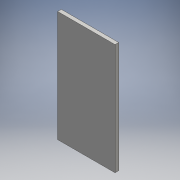
# Autodesk Inventor part: gora
Saved by Autodesk Inventor 2016 SP1 (Build 200210100, 210)
## iProperties
Created: 2019-02-20
Part Number: gora
Material: Ogólny
Document SubType Name: Modeling
Designer: Maciek
Density: 1 g/cm^3
Appearance: Domyślna
Author: Maciek
Autodesk Inventor part; units mm, degrees
ref_plane "YZ Plane" through (0, 0, 0) normal (1, 0, 0) x (0, 1, 0)
ref_plane "XZ Plane" through (0, 0, 0) normal (0, 1, 0) x (-1, 0, 0)
ref_plane "XY Plane" through (0, 0, 0) normal (0, 0, 1) x (1, 0, 0)
sketch "Szkic1" plane through (0, 0, 0) normal (0, 1, 0) x (-1, 0, 0)
  line L0 (0, 0) -> (23.5, 0)
  line L1 (23.5, 0) -> (23.5, 45.5)
  line L2 (23.5, 45.5) -> (0, 45.5)
  line L3 (0, 45.5) -> (0, 0)
  dimension "d0" = 23.5
  dimension "d1" = 45.5
  constraints: 8 end point, 2 parallel, 1 horizontal, 1 perpendicular
  measures "d0" distance of L2.end L1.end
  measures "d1" distance of L1.end L0.end
extrude "Wyciągnięcie proste1" add sketch "Szkic1" along normal blind 1.5
sketch "Szkic2" plane through (0, 1.5, 0) normal (0, 1, 0) x (1, 0, 0)
  line L0 (-23.5, 0) -> (-23.5, -45.5) construction
  line L1 (-23.5, -45.5) -> (-22, -45.5) construction
  line L2 (-23.5, -45.5) -> (0, -45.5) construction
  line L3 (-22, -45.5) -> (-22, -44) construction
  line L4 (-22, -44) -> (-1.5, -44)
  line L5 (-1.5, -44) -> (-1.5, -1.5)
  line L6 (-1.5, -1.5) -> (-22, -1.5)
  line L7 (-22, -1.5) -> (-22, -44)
  line L8 (-22, -44) -> (-22, -42.5) construction
  line L9 (-22, -42.5) -> (-20.5, -42.5) construction
  line L10 (-1.5, -1.5) -> (-3, -1.5) construction
  line L11 (-3, -1.5) -> (-3, -3) construction
  line L12 (-20.5, -42.5) -> (-3, -42.5)
  line L13 (-3, -42.5) -> (-3, -3)
  line L14 (-3, -3) -> (-20.5, -3)
  line L15 (-20.5, -3) -> (-20.5, -42.5)
  point P0 (0, 0)
  dimension "d4" = 1.5
  dimension "d5" = 1.5
  dimension "d6" = 20.5
  dimension "d7" = 42.5
  dimension "d8" = 1.5
  dimension "d9" = 1.5
  dimension "d10" = 1.5
  dimension "d11" = 1.5
  constraints: 28 end point, 4 parallel, 4 perpendicular, 3 point on line, 2 horizontal, 1 vertical
  measures "d4" distance of L0.end L1.end
  measures "d5" distance of L1.end L3.end
  measures "d6" distance of L6.end L5.end
  measures "d7" distance of L5.end L4.end
  measures "d8" distance of L3.end L8.end
  measures "d9" distance of L8.end L9.end
  measures "d10" distance of L5.end L10.end
  measures "d11" distance of L10.end L11.end
extrude "Wyciągnięcie proste2" add sketch "Szkic2" along normal blind 1.5
